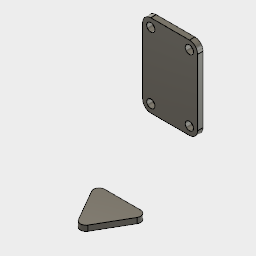
Course 2 Peer Review_ CSA011070 (Autodesk Fusion 360 design; units mm, degrees)
Autodesk Fusion 360 part; units mm, degrees
sketch "Sketch1" plane through (0, 0, 0) normal (0, 0, 1) x (1, 0, 0) in component "Mounting Plate1"
  line L0 (-50, 75) -> (50, 75)
  line L1 (50, 75) -> (50, -75)
  line L2 (50, -75) -> (-50, -75)
  line L3 (-50, -75) -> (-50, 75)
  line L4 (-50, 75) -> (50, -75) construction
  line L5 (50, 75) -> (-50, -75) construction
  circle A0 centre (-35, 60) radius 7.5
  circle A1 centre (35, 60) radius 7.5
  line L6 (0, 0) -> (21.7934, 0) construction
  circle A2 centre (-35, -60) radius 7.5
  circle A3 centre (35, -60) radius 7.5
  dimension "d1" = 100
  dimension "d2" = 150
  dimension "d3" = 15
  dimension "d4" = 15
  dimension "d5" = 15
  dimension "d6" = 15
  measures "d1" distance of L1.end L2.end
  measures "d2" distance of L0.end L1.end
  measures "d3" diameter of A1
  measures "d4" distance of L0 A1.centre
  measures "d5" distance of L1 A1.centre
  measures "d6" distance of L3 A0.centre
extrude "Extrude1" add sketch "Sketch1" along normal blind 10 makes body 1 in component "Mounting Plate1"
fillet "Fillet1" radius 15 4 edges at (-50, 75, 5) (50, 75, 5) (50, -75, 5) (-50, -75, 5) on bodies 1 in component "Mounting Plate1"
ref_plane "WorkPlane1" through (0, -150, 0) normal (0, 1, 0) x (0, 0, 1) in component "Mounting Plate1"
sketch "Sketch2" plane through (0, -150, 0) normal (0, 1, 0) x (1, 0, 0) in component "Mounting Plate1"
  line L0 (-35, -10) -> (35, -10)
  line L1 (0, 0) -> (0, -125) construction
  line L2 (-50, -96.1325) -> (0, -182.735)
  line L3 (0, -182.735) -> (50, -96.1325)
  line L4 (50, -96.1325) -> (-50, -96.1325)
  point P0 (0, -125)
  dimension "d11" = 125
  dimension "d12" = 100
  measures "d11" distance of L1.start P0
  measures "d12" distance of L2.start L3.end
extrude "Extrude2" add sketch "Sketch2" against normal blind 10 separate body makes body 2 in component "Mounting Plate1"
fillet "Fillet2" radius 10 3 edges at (0, -155, 182.735) (50, -155, 96.1325) (-50, -155, 96.1325) on bodies 2 in component "Mounting Plate1"
component "Mounting Plate1" placed x (1, 0, 0) y (0, 1, 0) z (0, 0, 1) at (0, 0, 0)
equation "d2 = ( 6 * 25 ) * 1 mm"
